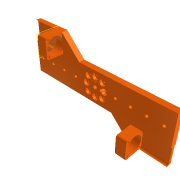
# Autodesk Inventor part: Gripper_linear_base
Saved by Autodesk Inventor 2022 (Build 260153000, 153)
## iProperties
Created: 2023-01-05
Part Number: Gripper_linear_base
Material: Generisch
Document SubType Name: Modeling
Designer: diederichbenedict
Density: 1 g/cm^3
Appearance: Glatt - Hellorange
Author: diederichbenedict
Autodesk Inventor part; units mm, degrees
ref_plane "YZ Plane" through (0, 0, 0) normal (1, 0, 0) x (0, 1, 0)
ref_plane "XZ Plane" through (0, 0, 0) normal (0, 1, 0) x (-1, 0, 0)
ref_plane "Arbeitsebene1" through (0, 0, 0) normal (0, 0, 1) x (1, 0, 0)
ref_plane "Arbeitsebene2" through (-62.5204, -6.05, 6) normal (0, 0, -1) x (0, 1, 0)
sketch "Skizze1" plane through (0, 0, 0) normal (0, 0, 1) x (1, 0, 0)
  arc A0 (2.6936, 12.5) -> (22.2655, 12.5) centre (12.4796, 0) ccw projected
  line L0 (2.6936, 12.5) -> (22.2655, 12.5) projected
  circle A1 centre (22.4796, 0) radius 1.2645 projected
  circle A2 centre (12.4796, -10) radius 1.2645 projected
  circle A3 centre (2.4796, 0) radius 1.2645 projected
  circle A4 centre (4.6218, 7.8577) radius 1.3843 projected
  circle A5 centre (20.3373, 7.8577) radius 1.3843 projected
  circle A6 centre (20.3373, -7.8577) radius 1.3843 projected
  circle A7 centre (4.6218, -7.8577) radius 1.3843 projected
  circle A8 centre (12.4796, 10) radius 1.2645 projected
  line L1 (15.8406, 4.9845) -> (16.6506, 4.9845) projected
  line L2 (15.8406, 5.2497) -> (15.8406, 4.9845) projected
  line L3 (16.6506, 5.2497) -> (15.8406, 5.2497) projected
  line L4 (16.6506, 4.9845) -> (16.6506, 5.2497) projected
  spline S0 degree 3 poles (11.8122, 3.7087) (11.8794, 3.7128) (12.0048, 3.7206) (12.0893, 3.8125) (12.1286, 3.8551) knots 0 0 0 0 0.01932 0.036091 0.036091 0.036091 0.036091 projected
  spline S1 degree 3 poles (11.6057, 3.7365) (11.6393, 3.7284) (11.7072, 3.712) (11.777, 3.7098) (11.8122, 3.7087) knots 0 0 0 0 0.010357 0.02089 0.02089 0.02089 0.02089 projected
  line L5 (11.6555, 3.9606) -> (11.6057, 3.7365) projected
  spline S2 degree 3 poles (11.78, 3.9401) (11.762, 3.9414) (11.7199, 3.9443) (11.6789, 3.9547) (11.6555, 3.9606) knots 0 0 0 0 0.005408 0.012641 0.012641 0.012641 0.012641 projected
  spline S3 degree 3 poles (11.9001, 3.9936) (11.8845, 3.978) (11.8515, 3.945) (11.8047, 3.9418) (11.78, 3.9401) knots 0 0 0 0 0.006394 0.013551 0.013551 0.013551 0.013551 projected
  spline S4 degree 3 poles (11.9397, 4.2609) (11.9409, 4.2021) (11.9429, 4.1102) (11.9115, 4.0245) (11.9001, 3.9936) knots 0 0 0 0 0.017405 0.02722 0.02722 0.02722 0.02722 projected
  line L6 (11.9397, 5.8957) -> (11.9397, 4.2609) projected
  line L7 (12.2033, 5.8957) -> (11.9397, 5.8957) projected
  line L8 (12.2033, 4.255) -> (12.2033, 5.8957) projected
  spline S5 degree 3 poles (12.1286, 3.8551) (12.1502, 3.9066) (12.2036, 4.0339) (12.2034, 4.1725) (12.2033, 4.255) knots 0 0 0 0 0.016611 0.041035 0.041035 0.041035 0.041035 projected
  line L9 (9.0759, 4.6872) -> (9.3249, 4.6872) projected
  line L10 (9.0759, 5.276) -> (9.0759, 4.6872) projected
  line L11 (8.4914, 5.276) -> (9.0759, 5.276) projected
  line L12 (8.4914, 5.5221) -> (8.4914, 5.276) projected
  line L13 (9.0759, 5.5221) -> (8.4914, 5.5221) projected
  line L14 (9.0759, 6.1066) -> (9.0759, 5.5221) projected
  line L15 (9.3249, 6.1066) -> (9.0759, 6.1066) projected
  line L16 (9.3249, 5.5221) -> (9.3249, 6.1066) projected
  line L17 (9.9094, 5.5221) -> (9.3249, 5.5221) projected
  line L18 (9.9094, 5.276) -> (9.9094, 5.5221) projected
  line L19 (9.3249, 5.276) -> (9.9094, 5.276) projected
  line L20 (9.3249, 4.6872) -> (9.3249, 5.276) projected
  line L21 (11.9397, 6.1813) -> (12.2033, 6.1813) projected
  line L22 (11.9397, 6.4875) -> (11.9397, 6.1813) projected
  line L23 (12.2033, 6.4875) -> (11.9397, 6.4875) projected
  line L24 (12.2033, 6.1813) -> (12.2033, 6.4875) projected
  line L25 (13.3796, 4.34) -> (13.6433, 4.34) projected
  line L26 (13.3796, 4.8542) -> (13.3796, 4.34) projected
  line L27 (12.448, 4.8542) -> (13.3796, 4.8542) projected
  line L28 (12.448, 5.0959) -> (12.448, 4.8542) projected
  line L29 (13.428, 6.4875) -> (12.448, 5.0959) projected
  line L30 (13.6433, 6.4875) -> (13.428, 6.4875) projected
  line L31 (13.6433, 5.0959) -> (13.6433, 6.4875) projected
  line L32 (13.9333, 5.0959) -> (13.6433, 5.0959) projected
  line L33 (13.9333, 4.8542) -> (13.9333, 5.0959) projected
  line L34 (13.6433, 4.8542) -> (13.9333, 4.8542) projected
  line L35 (13.6433, 4.34) -> (13.6433, 4.8542) projected
  circle A9 centre (12.4796, 0) radius 2 projected
  line L36 (-62.5204, -6.05) -> (87.4796, -6.05) projected
  line L37 (-62.5204, 6.05) -> (87.4796, 6.05) projected
  line L38 (86.9796, -36.25) -> (61.0796, -36.25) projected
  line L39 (61.0796, -16.05) -> (86.9796, -16.05) projected
  line L40 (-36.1204, 16.05) -> (-62.0204, 16.05) projected
  line L41 (87.4796, -16.05) -> (-62.0204, -16.05)
  line L42 (-62.0204, -16.05) -> (-62.0204, 16.05)
  line L43 (-62.0204, 16.05) -> (87.4796, 16.05)
  line L44 (87.4796, 16.05) -> (87.4796, -16.05)
  point P0 (0, 0)
  constraints: 8 end point, 2 parallel, 2 point on line, 1 horizontal, 1 perpendicular
extrude "Extrusion1" add sketch "Skizze1" along normal up to surface (6 mm away) contours L0 A0 L37 L31 L30 L29 L16 L15 L14 | A0 L37 L42 L40 L43 L44 L0 | L37 L14 L13 L12 L11 L10 L9 L20 L19 L18 L17 L16 L29 L28 L27 L26 L25 L35 L34 L33 L32 L31 A0 L36 | A0 L36 L42 L37 | L36 A0 | A0 L36 L44 L41 L39 L42 | L37 L44 L36 A0
ref_plane "Arbeitsebene3" through (-36.1204, 16.05, 3) normal (1, 0, 0) x (0, 1, 0)
sketch "Skizze2" plane through (-36.1204, 16.05, 3) normal (1, 0, 0) x (0, 1, 0)
  line L0 (0, 17.9) -> (0, 2.3) projected
  arc A0 (0, 2.3) -> (2.3, 0) centre (2.3, 2.3) ccw projected
  line L1 (2.3, 0) -> (17.9, 0) projected
  arc A1 (17.9, 0) -> (20.2, 2.3) centre (17.9, 2.3) ccw projected
  line L2 (20.2, 2.3) -> (20.2, 17.9) projected
  arc A2 (20.2, 17.9) -> (17.9, 20.2) centre (17.9, 17.9) ccw projected
  line L3 (17.9, 20.2) -> (2.3, 20.2) projected
  arc A3 (2.3, 20.2) -> (0, 17.9) centre (2.3, 17.9) ccw projected
  circle A4 centre (10.1, 10.1) radius 8 projected
  circle A5 centre (2.4, 2.4) radius 1 projected
  circle A6 centre (17.8, 2.4) radius 1 projected
  circle A7 centre (17.8, 17.8) radius 1 projected
  circle A8 centre (2.4, 17.8) radius 1 projected
  circle A9 centre (10.1, 10.1) radius 9
  line L4 (0, -3) -> (0, 3) projected
  line L5 (20.2, 2.3) -> (20.2, -3)
  line L6 (20.2, -3) -> (0, -3)
  line L7 (0, -3) -> (0, 2.3)
  line L8 (0, 2.3) -> (1.405, 2.3)
  line L9 (3.395, 2.3) -> (16.805, 2.3)
  line L10 (18.795, 2.3) -> (20.2, 2.3)
  point P0 (-16.05, -3)
  point P1 (20.2, 2.3)
  dimension "d2" = 18
  constraints: 12 end point, 5 point on circle, 4 parallel, 3 horizontal, 3 perpendicular, 1 centre point, 1 coincident, 1 point on line
  measures "d2" diameter of A9
extrude "Extrusion2" add sketch "Skizze2" along normal blind 10 contours A3 L3 A2 L2 L10 A6 L9 A9 A5 L8 L0 | L8 A5 L9 A9 A6 L10 A1 L1 A0 | A0 L1 A1 L5 L6 L4
sketch "Skizze3" plane through (-36.1204, 16.05, 3) normal (-1, 0, 0) x (0, 0, 1)
  arc A0 (2.3, 20.2) -> (0, 17.9) centre (2.3, 17.9) ccw projected
  line L0 (0, 14.9) -> (0, 17.9) projected
  line L1 (0, 5.3) -> (0, 14.9) projected
  line L2 (0, 2.3) -> (0, 5.3) projected
  arc A1 (0, 2.3) -> (2.3, 0) centre (2.3, 2.3) ccw projected
  line L3 (17.9, 0) -> (3, 0) projected
  arc A2 (17.9, 0) -> (20.2, 2.3) centre (17.9, 2.3) ccw projected
  line L4 (20.2, 17.9) -> (20.2, 2.3) projected
  arc A3 (20.2, 17.9) -> (17.9, 20.2) centre (17.9, 17.9) ccw projected
  line L5 (-3, 20.2) -> (17.9, 20.2) projected
  line L6 (-3, 0) -> (-3, 20.2) projected
  line L7 (3, 0) -> (-3, 0) projected
  circle A4 centre (10.1, 10.1) radius 9 projected
  circle A5 centre (17.8, 2.4) radius 1 projected
  circle A6 centre (17.8, 17.8) radius 1 projected
  circle A7 centre (2.4, 17.8) radius 1 projected
  circle A8 centre (2.4, 2.4) radius 1 projected
  point P0 (-3, -16.05)
  point P1 (2.3, 20.2)
  point P2 (2.3, 0)
extrude "Extrusion3" add sketch "Skizze3" along normal up to surface (25.9 mm away) contours A0 L0 L1 L2 A1 L7 L6 L5
pattern_circular "Runde Anordnung1" count 2 over 360 about axis through (12.4796, 0, 0) along (0, 0, 1) of "Extrusion2", "Extrusion3"
sketch "Skizze4" plane through (87.4796, -16.05, 6) normal (0, 0, 1) x (1, 0, 0)
  line L0 (0, 0) -> (0, 32.1) projected
  line L1 (0, 32.1) -> (-113.6, 32.1) projected
  line L2 (-113.6, 32.1) -> (-123.6, 32.1) projected
  line L3 (-123.6, 32.1) -> (-149.5, 32.1) projected
  line L4 (-149.5, 32.1) -> (-149.5, 0) projected
  line L5 (-149.5, 0) -> (-36.4, 0) projected
  line L6 (-36.4, 0) -> (-26.4, 0) projected
  line L7 (-26.4, 0) -> (0, 0) projected
  circle A0 centre (-82.8577, 8.1923) radius 1.3843 projected
  circle A1 centre (-67.1423, 8.1923) radius 1.3843 projected
  circle A2 centre (-75, 6.05) radius 1.2645 projected
  line L8 (-74.0516, 22.5375) -> (-73.8363, 22.5375) projected
  line L9 (-73.8363, 22.5375) -> (-73.8363, 21.1459) projected
  line L10 (-73.8363, 21.1459) -> (-73.5462, 21.1459) projected
  line L11 (-73.5462, 21.1459) -> (-73.5462, 20.9042) projected
  line L12 (-73.5462, 20.9042) -> (-73.8363, 20.9042) projected
  line L13 (-73.8363, 20.9042) -> (-73.8363, 20.39) projected
  line L14 (-73.8363, 20.39) -> (-74.0999, 20.39) projected
  line L15 (-74.0999, 20.39) -> (-74.0999, 20.9042) projected
  line L16 (-74.0999, 20.9042) -> (-75.0316, 20.9042) projected
  line L17 (-75.0316, 20.9042) -> (-75.0316, 21.1459) projected
  line L18 (-75.0316, 21.1459) -> (-74.0516, 22.5375) projected
  line L19 (-78.4037, 22.1566) -> (-78.1546, 22.1566) projected
  line L20 (-78.1546, 22.1566) -> (-78.1546, 21.5721) projected
  line L21 (-78.1546, 21.5721) -> (-77.5702, 21.5721) projected
  line L22 (-77.5702, 21.5721) -> (-77.5702, 21.326) projected
  line L23 (-77.5702, 21.326) -> (-78.1546, 21.326) projected
  line L24 (-78.1546, 21.326) -> (-78.1546, 20.7372) projected
  line L25 (-78.1546, 20.7372) -> (-78.4037, 20.7372) projected
  line L26 (-78.4037, 20.7372) -> (-78.4037, 21.326) projected
  line L27 (-78.4037, 21.326) -> (-78.9881, 21.326) projected
  line L28 (-78.9881, 21.326) -> (-78.9881, 21.5721) projected
  line L29 (-78.9881, 21.5721) -> (-78.4037, 21.5721) projected
  line L30 (-78.4037, 21.5721) -> (-78.4037, 22.1566) projected
  line L31 (-75.2762, 22.2313) -> (-75.5399, 22.2313) projected
  line L32 (-75.5399, 22.2313) -> (-75.5399, 22.5375) projected
  line L33 (-75.5399, 22.5375) -> (-75.2762, 22.5375) projected
  line L34 (-75.2762, 22.5375) -> (-75.2762, 22.2313) projected
  circle A3 centre (-75, 26.05) radius 1.2645 projected
  circle A4 centre (-67.1423, 23.9077) radius 1.3843 projected
  circle A5 centre (-82.8577, 23.9077) radius 1.3843 projected
  circle A6 centre (-75, 16.05) radius 2 projected
  line L35 (-75.8739, 19.7865) -> (-75.8241, 20.0106) projected
  line L36 (-75.5399, 20.3109) -> (-75.5399, 21.9457) projected
  line L37 (-75.5399, 21.9457) -> (-75.2762, 21.9457) projected
  line L38 (-75.2762, 21.9457) -> (-75.2762, 20.305) projected
  line L39 (-70.8289, 21.0345) -> (-71.639, 21.0345) projected
  line L40 (-71.639, 21.0345) -> (-71.639, 21.2997) projected
  line L41 (-71.639, 21.2997) -> (-70.8289, 21.2997) projected
  line L42 (-70.8289, 21.2997) -> (-70.8289, 21.0345) projected
  circle A7 centre (-85, 16.05) radius 1.2645 projected
  circle A8 centre (-65, 16.05) radius 1.2645 projected
  point P0 (-87.4796, 16.05)
  point P1 (-75.3509, 19.9051)
  point P2 (-75.6673, 19.7587)
  point P3 (-75.6996, 19.9901)
  point P4 (-75.5794, 20.0436)
  constraints: 6 other
hole "Bohrung1" at (20.3373, -7.8577, 6) at (12.4796, -10, 6) at (4.6218, -7.8577, 6) at (2.4796, 0, 6) at (4.6218, 7.8577, 6) at (12.4796, 10, 6) at (20.3373, 7.8577, 6) at (22.4796, 0, 6) direction (0, 0, -1) diameter 3 end through all counterbore diameter 6.5 counterbore depth 3
sketch "Skizze5" plane through (0, 0, 0) normal (0, 0, -1) x (-1, 0, 0)
  circle A0 centre (-79.3812, 0.1) radius 1.75 projected
  point P0 (0, 0)
hole "Bohrung2" at (79.3812, 0.1, 0) direction (0, 0, 1) diameter 3 end through all counterbore diameter 6.5 counterbore depth 3
pattern_linear "Rechteckige Anordnung1" count 10 spacing 15 along (-1, 0, 0) of "Bohrung2"
sketch "Skizze6" plane through (0, 0, 0) normal (0, 0, -1) x (-1, 0, 0)
  line L0 (-15.8406, 4.9845) -> (-15.8406, 5.2497) projected
  line L1 (-16.6506, 4.9845) -> (-15.8406, 4.9845) projected
  line L2 (-16.6506, 5.2497) -> (-16.6506, 4.9845) projected
  line L3 (-15.8406, 5.2497) -> (-16.6506, 5.2497) projected
  line L4 (-12.2033, 5.8957) -> (-12.2033, 4.255) projected
  line L5 (-11.9397, 5.8957) -> (-12.2033, 5.8957) projected
  line L6 (-11.9397, 4.2609) -> (-11.9397, 5.8957) projected
  line L7 (-11.6057, 3.7365) -> (-11.6555, 3.9606) projected
  circle A0 centre (-12.4796, 0) radius 2 projected
  line L8 (-11.9397, 6.1813) -> (-11.9397, 6.4875) projected
  line L9 (-12.2033, 6.1813) -> (-11.9397, 6.1813) projected
  line L10 (-12.2033, 6.4875) -> (-12.2033, 6.1813) projected
  line L11 (-11.9397, 6.4875) -> (-12.2033, 6.4875) projected
  line L12 (-9.3249, 6.1066) -> (-9.3249, 5.5221) projected
  line L13 (-9.0759, 6.1066) -> (-9.3249, 6.1066) projected
  line L14 (-9.0759, 5.5221) -> (-9.0759, 6.1066) projected
  line L15 (-8.4914, 5.5221) -> (-9.0759, 5.5221) projected
  line L16 (-8.4914, 5.276) -> (-8.4914, 5.5221) projected
  line L17 (-9.0759, 5.276) -> (-8.4914, 5.276) projected
  line L18 (-9.0759, 4.6872) -> (-9.0759, 5.276) projected
  line L19 (-9.3249, 4.6872) -> (-9.0759, 4.6872) projected
  line L20 (-9.3249, 5.276) -> (-9.3249, 4.6872) projected
  line L21 (-9.9094, 5.276) -> (-9.3249, 5.276) projected
  line L22 (-9.9094, 5.5221) -> (-9.9094, 5.276) projected
  line L23 (-9.3249, 5.5221) -> (-9.9094, 5.5221) projected
  line L24 (-13.6433, 6.4875) -> (-13.6433, 5.0959) projected
  line L25 (-13.428, 6.4875) -> (-13.6433, 6.4875) projected
  line L26 (-12.448, 5.0959) -> (-13.428, 6.4875) projected
  line L27 (-12.448, 4.8542) -> (-12.448, 5.0959) projected
  line L28 (-13.3796, 4.8542) -> (-12.448, 4.8542) projected
  line L29 (-13.3796, 4.34) -> (-13.3796, 4.8542) projected
  line L30 (-13.6433, 4.34) -> (-13.3796, 4.34) projected
  line L31 (-13.6433, 4.8542) -> (-13.6433, 4.34) projected
  line L32 (-13.9333, 4.8542) -> (-13.6433, 4.8542) projected
  line L33 (-13.9333, 5.0959) -> (-13.9333, 4.8542) projected
  line L34 (-13.6433, 5.0959) -> (-13.9333, 5.0959) projected
  line L35 (-87.4796, 16.05) -> (26.1204, 16.05) projected
  line L36 (-87.4796, -16.05) -> (-87.4796, 16.05) projected
  line L37 (-86.9796, -16.05) -> (-87.4796, -16.05) projected
  line L38 (-86.9796, -16.05) -> (-86.9796, -36.25) projected
  line L39 (-86.9796, -36.25) -> (-51.0796, -36.25) projected
  line L40 (-51.0796, -16.05) -> (-51.0796, -36.25) projected
  line L41 (62.0204, -16.05) -> (-51.0796, -16.05) projected
  line L42 (62.0204, -16.05) -> (62.0204, 36.25) projected
  line L43 (62.0204, 36.25) -> (26.1204, 36.25) projected
  line L44 (26.1204, 16.05) -> (26.1204, 36.25) projected
  arc A1 (-22.2225, -1.4778) -> (-22.3184, 1.4913) centre (-19.3812, 0.1) ccw projected
  arc A2 (-22.3184, 1.4913) -> (-22.2225, -1.4778) centre (-22.4796, 0) ccw projected
  circle A3 centre (-12.4796, 10) radius 1.5 projected
  circle A4 centre (-12.4796, -10) radius 1.5 projected
  circle A5 centre (-20.3373, -7.8577) radius 1.5 projected
  circle A6 centre (-4.6218, -7.8577) radius 1.5 projected
  circle A7 centre (-4.6218, 7.8577) radius 1.5 projected
  circle A8 centre (-20.3373, 7.8577) radius 1.5 projected
  circle A9 centre (-79.3812, 0.1) radius 3.25 projected
  circle A10 centre (-64.3812, 0.1) radius 3.25 projected
  circle A11 centre (-49.3812, 0.1) radius 3.25 projected
  circle A12 centre (-34.3812, 0.1) radius 3.25 projected
  circle A13 centre (10.6188, 0.1) radius 3.25 projected
  circle A14 centre (25.6188, 0.1) radius 3.25 projected
  circle A15 centre (40.6188, 0.1) radius 3.25 projected
  circle A16 centre (55.6188, 0.1) radius 3.25 projected
  arc A17 (-1.2058, 0.7921) -> (-1.2959, -0.9214) centre (-4.3812, 0.1) ccw projected
  arc A18 (-1.2959, -0.9214) -> (-1.2058, 0.7921) centre (-2.4796, 0) ccw projected
  line L45 (-86.9796, -36.25) -> (-51.0796, -36.25) projected
  line L46 (-51.0796, -36.25) -> (-30.8796, -16.05)
  line L47 (62.0204, -16.05) -> (-51.0796, -16.05) projected
  line L48 (-51.0796, -36.25) -> (-22.5124, -36.25) construction
  line L49 (26.1204, 16.05) -> (26.1204, 36.25) projected
  line L50 (26.1204, 36.25) -> (5.9204, 16.05)
  line L51 (-87.4796, 16.05) -> (26.1204, 16.05) projected
  line L52 (26.1204, 36.25) -> (54.6876, 36.25) construction
  point P0 (0, 0)
  point P1 (-11.8122, 3.7087)
  point P2 (-12.1286, 3.8551)
  point P3 (-11.9001, 3.9936)
  point P4 (-11.78, 3.9401)
  point P5 (-30.8796, -16.05)
  point P6 (5.9204, 16.05)
  dimension "d27" = 45
  dimension "d28" = 135
  constraints: 8 end point, 2 equal length, 2 horizontal, 2 point on line, 6 other
  measures "d27" angle of L48 L46
  measures "d28" angle of L50 L52
extrude "Extrusion4" add sketch "Skizze6" against normal up to surface (6 mm away) contours L50 L44 L35 | L40 L41 L46
